Autodesk Fusion 360 part; units mm, degrees
(part 3 of 4)
sketch "Sketch6" plane through (0, 0, 4.8) normal (0, 0, 1) x (-1, 0, 0)
  circle A0 centre (64.2941, -62.4) radius 1.5
  circle A1 centre (64.2941, 62.4) radius 1.5
  circle A2 centre (97.2941, -62.4) radius 1.5
  circle A3 centre (97.2941, 62.4) radius 1.5
  circle A4 centre (1.7941, -104.2) radius 6.1
  line L0 (15.4941, 111.4) -> (41.8941, 111.4)
  arc A5 (45.5941, 107.7) -> (41.8941, 111.4) centre (41.8941, 107.7) ccw
  line L1 (45.5941, 107.7) -> (45.5941, 100.7)
  arc A6 (41.8941, 97) -> (45.5941, 100.7) centre (41.8941, 100.7) ccw
  line L2 (41.8941, 97) -> (15.4941, 97)
  arc A7 (11.7941, 100.7) -> (15.4941, 97) centre (15.4941, 100.7) ccw
  line L3 (11.7941, 100.7) -> (11.7941, 107.7)
  arc A8 (15.4941, 111.4) -> (11.7941, 107.7) centre (15.4941, 107.7) ccw
  line L4 (15.4941, -97) -> (41.8941, -97)
  arc A9 (45.5941, -100.7) -> (41.8941, -97) centre (41.8941, -100.7) ccw
  line L5 (45.5941, -100.7) -> (45.5941, -107.7)
  arc A10 (41.8941, -111.4) -> (45.5941, -107.7) centre (41.8941, -107.7) ccw
  line L6 (41.8941, -111.4) -> (15.4941, -111.4)
  arc A11 (11.7941, -107.7) -> (15.4941, -111.4) centre (15.4941, -107.7) ccw
  line L7 (11.7941, -107.7) -> (11.7941, -100.7)
  arc A12 (15.4941, -97) -> (11.7941, -100.7) centre (15.4941, -100.7) ccw
  circle A13 centre (45.4941, 42.5) radius 1.5
  arc A14 (94.6728, -10) -> (96.7941, -7.8787) centre (95.7335, -8.9393) ccw
  line L8 (94.6728, -10) -> (94.1155, -10)
  arc A15 (91.9941, -7.8787) -> (94.1155, -10) centre (93.0548, -8.9393) ccw
  line L9 (91.9941, -7.8787) -> (91.9941, 7.8787)
  arc A16 (94.1155, 10) -> (91.9941, 7.8787) centre (93.0548, 8.9393) ccw
  line L10 (94.1155, 10) -> (94.6728, 10)
  arc A17 (96.7941, 7.8787) -> (94.6728, 10) centre (95.7335, 8.9393) ccw
  line L11 (96.7941, 7.8787) -> (96.7941, -7.8787)
  arc A18 (39.8728, -10) -> (41.9941, -7.8787) centre (40.9335, -8.9393) ccw
  line L12 (39.8728, -10) -> (39.3155, -10)
  arc A19 (37.1941, -7.8787) -> (39.3155, -10) centre (38.2548, -8.9393) ccw
  line L13 (37.1941, -7.8787) -> (37.1941, 7.8787)
  arc A20 (39.3155, 10) -> (37.1941, 7.8787) centre (38.2548, 8.9393) ccw
  line L14 (39.3155, 10) -> (39.8728, 10)
  arc A21 (41.9941, 7.8787) -> (39.8728, 10) centre (40.9335, 8.9393) ccw
  line L15 (41.9941, 7.8787) -> (41.9941, -7.8787)
  circle A22 centre (-123.5112, 37.2289) radius 1.5
  circle A23 centre (64.5, 111.7173) radius 1.5
  arc A24 (-55.2202, 79.8868) -> (-55.9967, 76.9891) centre (-55.6084, 78.438) ccw
  line L16 (-55.2202, 79.8868) -> (-41.5739, 87.7655)
  arc A25 (-38.6762, 86.9891) -> (-41.5739, 87.7655) centre (-40.125, 87.3773) ccw
  line L17 (-38.6762, 86.9891) -> (-38.3975, 86.5064)
  arc A26 (-39.1739, 83.6086) -> (-38.3975, 86.5064) centre (-38.7857, 85.0575) ccw
  line L18 (-39.1739, 83.6086) -> (-52.8202, 75.7299)
  arc A27 (-55.718, 76.5064) -> (-52.8202, 75.7299) centre (-54.2691, 76.1181) ccw
  line L19 (-55.718, 76.5064) -> (-55.9967, 76.9891)
  circle A28 centre (-123.5112, -37.2289) radius 1.5
  circle A29 centre (64.5, -111.7173) radius 1.5
  arc A30 (-11.2762, 39.5309) -> (-14.1739, 40.3073) centre (-12.725, 39.9191) ccw
  line L20 (-11.2762, 39.5309) -> (-10.9975, 39.0482)
  arc A31 (-11.7739, 36.1504) -> (-10.9975, 39.0482) centre (-11.3857, 37.5993) ccw
  line L21 (-11.7739, 36.1504) -> (-25.4202, 28.2717)
  arc A32 (-28.318, 29.0482) -> (-25.4202, 28.2717) centre (-26.8691, 28.66) ccw
  line L22 (-28.318, 29.0482) -> (-28.5967, 29.5309)
  arc A33 (-27.8202, 32.4286) -> (-28.5967, 29.5309) centre (-28.2084, 30.9798) ccw
  line L23 (-27.8202, 32.4286) -> (-14.1739, 40.3073)
  arc A34 (-10.9975, -39.0482) -> (-11.7739, -36.1504) centre (-11.3857, -37.5993) ccw
  line L24 (-10.9975, -39.0482) -> (-11.2762, -39.5309)
  arc A35 (-14.1739, -40.3073) -> (-11.2762, -39.5309) centre (-12.725, -39.9191) ccw
  line L25 (-14.1739, -40.3073) -> (-27.8202, -32.4286)
  arc A36 (-28.5967, -29.5309) -> (-27.8202, -32.4286) centre (-28.2084, -30.9798) ccw
  line L26 (-28.5967, -29.5309) -> (-28.318, -29.0482)
  arc A37 (-25.4202, -28.2717) -> (-28.318, -29.0482) centre (-26.8691, -28.66) ccw
  line L27 (-25.4202, -28.2717) -> (-11.7739, -36.1504)
  arc A38 (-52.8202, -75.7299) -> (-55.718, -76.5064) centre (-54.2691, -76.1181) ccw
  line L28 (-52.8202, -75.7299) -> (-39.1739, -83.6086)
  arc A39 (-38.3975, -86.5064) -> (-39.1739, -83.6086) centre (-38.7857, -85.0575) ccw
  line L29 (-38.3975, -86.5064) -> (-38.6762, -86.9891)
  arc A40 (-41.5739, -87.7655) -> (-38.6762, -86.9891) centre (-40.125, -87.3773) ccw
  line L30 (-41.5739, -87.7655) -> (-55.2202, -79.8868)
  arc A41 (-55.9967, -76.9891) -> (-55.2202, -79.8868) centre (-55.6084, -78.438) ccw
  line L31 (-55.9967, -76.9891) -> (-55.718, -76.5064)
  circle A42 centre (45.4941, -42.5) radius 1.5
  line L32 (-42.1213, -25.5) -> (-109.5263, -25.5)
  arc A43 (-109.5263, -25.5) -> (-110.7763, -25.8349) centre (-109.5263, -28) ccw
  line L33 (-110.7763, -25.8349) -> (-125.9451, -34.5927)
  arc A44 (-125.9451, -34.5927) -> (-127.0931, -37.4646) centre (-124.6951, -36.7577) ccw
  arc A45 (-127.0931, -37.4646) -> (-89.0244, -98.1371) centre (0, 0) ccw
  arc A46 (-89.0244, -98.1371) -> (-85.1797, -97.5355) centre (-87.3447, -96.2855) ccw
  line L34 (-85.1797, -97.5355) -> (-74.6084, -79.2255)
  arc A47 (-71.7106, -78.449) -> (-74.6084, -79.2255) centre (-73.1595, -78.8372) ccw
  line L35 (-71.7106, -78.449) -> (-32.0836, -101.3277)
  arc A48 (-31.3071, -104.2255) -> (-32.0836, -101.3277) centre (-31.6953, -102.7766) ccw
  line L36 (-31.3071, -104.2255) -> (-41.8784, -122.5355)
  arc A49 (-41.8784, -122.5355) -> (-40.477, -126.166) centre (-39.7133, -123.7855) ccw
  arc A50 (-40.477, -126.166) -> (129.5015, -28.0288) centre (0, 0) ccw
  arc A51 (129.5015, -28.0288) -> (127.0581, -25) centre (127.0581, -27.5) ccw
  line L37 (127.0581, -25) -> (105.9155, -25)
  arc A52 (103.7941, -22.8787) -> (105.9155, -25) centre (104.8548, -23.9393) ccw
  line L38 (103.7941, -22.8787) -> (103.7941, 22.8787)
  arc A53 (105.9155, 25) -> (103.7941, 22.8787) centre (104.8548, 23.9393) ccw
  line L39 (105.9155, 25) -> (127.0581, 25)
  arc A54 (127.0581, 25) -> (129.5015, 28.0288) centre (127.0581, 27.5) ccw
  arc A55 (129.5015, 28.0288) -> (-40.477, 126.166) centre (0, 0) ccw
  arc A56 (-40.477, 126.166) -> (-41.8784, 122.5355) centre (-39.7133, 123.7855) ccw
  line L40 (-41.8784, 122.5355) -> (-31.3071, 104.2255)
  arc A57 (-32.0836, 101.3277) -> (-31.3071, 104.2255) centre (-31.6953, 102.7766) ccw
  line L41 (-32.0836, 101.3277) -> (-71.7106, 78.449)
  arc A58 (-74.6084, 79.2255) -> (-71.7106, 78.449) centre (-73.1595, 78.8372) ccw
  line L42 (-74.6084, 79.2255) -> (-85.1797, 97.5355)
  arc A59 (-85.1797, 97.5355) -> (-89.0244, 98.1371) centre (-87.3447, 96.2855) ccw
  arc A60 (-89.0244, 98.1371) -> (-127.0931, 37.4646) centre (0, 0) ccw
  arc A61 (-127.0931, 37.4646) -> (-125.9451, 34.5927) centre (-124.6951, 36.7577) ccw
  line L43 (-125.9451, 34.5927) -> (-110.7763, 25.8349)
  arc A62 (-110.7763, 25.8349) -> (-109.5263, 25.5) centre (-109.5263, 28) ccw
  line L44 (-109.5263, 25.5) -> (-42.1213, 25.5)
  arc A63 (-40, 23.3787) -> (-42.1213, 25.5) centre (-41.0607, 24.4393) ccw
  line L45 (-40, 23.3787) -> (-40, 20.8)
  arc A64 (-40, 20.8) -> (-37.5, 18.3) centre (-37.5, 20.8) ccw
  line L46 (-37.5, 18.3) -> (-34.1213, 18.3)
  arc A65 (-32, 16.1787) -> (-34.1213, 18.3) centre (-33.0607, 17.2393) ccw
  line L47 (-32, 16.1787) -> (-32, -16.1787)
  arc A66 (-34.1213, -18.3) -> (-32, -16.1787) centre (-33.0607, -17.2393) ccw
  line L48 (-34.1213, -18.3) -> (-37.5, -18.3)
  arc A67 (-37.5, -18.3) -> (-40, -20.8) centre (-37.5, -20.8) ccw
  line L49 (-40, -20.8) -> (-40, -23.3787)
  arc A68 (-42.1213, -25.5) -> (-40, -23.3787) centre (-41.0607, -24.4393) ccw
  arc A69 (-40.477, -126.166) -> (129.5015, -28.0288) centre (0, 0) ccw
  line L50 (57.7941, -64.8) -> (103.7941, -64.8)
  line L51 (57.7941, -58.1213) -> (57.7941, -83.8787)
  arc A70 (129.5015, 28.0288) -> (-40.477, 126.166) centre (0, 0) ccw
  line L52 (57.7941, 64.8) -> (103.7941, 64.8)
  line L53 (57.7941, 58.1213) -> (57.7941, 83.8787)
  line L54 (95.1844, -72.8) -> (67.2941, -72.8)
  line L55 (65.7941, -74.3) -> (65.7941, -100.26)
  arc A71 (68.1301, -101.5054) -> (96.3668, -75.223) centre (0, 0) ccw
  arc A72 (67.2941, -72.8) -> (65.7941, -74.3) centre (67.2941, -74.3) ccw
  arc A73 (65.7941, -100.26) -> (68.1301, -101.5054) centre (67.2941, -100.26) ccw
  arc A74 (96.3668, -75.223) -> (95.1844, -72.8) centre (95.1844, -74.3) ccw
  line L56 (95.1844, 72.8) -> (67.2941, 72.8)
  line L57 (65.7941, 74.3) -> (65.7941, 100.26)
  arc A75 (96.3668, 75.223) -> (68.1301, 101.5054) centre (0, 0) ccw
  arc A76 (65.7941, 74.3) -> (67.2941, 72.8) centre (67.2941, 74.3) ccw
  arc A77 (95.1844, 72.8) -> (96.3668, 75.223) centre (95.1844, 74.3) ccw
  arc A78 (68.1301, 101.5054) -> (65.7941, 100.26) centre (67.2941, 100.26) ccw
  circle A79 centre (-94.9024, 87.3758) radius 1.5
  circle A80 centre (123.1209, -38.5) radius 1.5
  circle A81 centre (123.1209, 38.5) radius 1.5
  circle A82 centre (-28.2185, 125.8758) radius 1.5
  circle A83 centre (-94.9024, -87.3758) radius 1.5
  circle A84 centre (-28.2185, -125.8758) radius 1.5
  dimension "d304" = 8
  dimension "d305" = 8
  dimension "d306" = 122.25
  dimension "d307" = 1.5
  dimension "d308" = 1.5
  dimension "d309" = 1.5
  dimension "d310" = 8
  dimension "d311" = 8
  dimension "d312" = 122.25
  dimension "d313" = 1.5
  dimension "d314" = 1.5
  dimension "d315" = 1.5
  constraint perpendicular L51 L54
  constraint perpendicular L54 L55
  constraint coincident A45.centre A50.centre
  constraint tangent L54 A72
  constraint tangent L55 A72
  constraint tangent A71 A73
  constraint tangent L55 A73
  constraint tangent A71 A74
  constraint tangent L54 A74
  constraint perpendicular L53 L56
  constraint perpendicular L56 L57
  constraint tangent L56 A76
  constraint tangent L57 A76
  constraint tangent A75 A77
  constraint tangent L56 A77
  constraint tangent A75 A78
  constraint tangent L57 A78
  measures "d304" distance of L50 L54
  measures "d305" distance of L51 L55
  measures "d306" radius of A71
  measures "d307" radius of A72
  measures "d308" radius of A73
  measures "d309" radius of A74
  measures "d310" distance of L52 L56
  measures "d311" distance of L53 L57
  measures "d312" radius of A75
  measures "d313" radius of A76
  measures "d314" radius of A77
  measures "d315" radius of A78
extrude "Extrude9" cut sketch "Sketch6" against normal through all contours L54 L55 A71 A72 A73 A74 | L56 L57 A75 A76 A77 A78
sketch "Sketch7" plane through (0, 0, 4.8) normal (0, 0, 1) x (-1, 0, 0)
  line L0 (11.7941, 92) -> (48.7941, 92)
  line L1 (11.7941, 89.8787) -> (11.7941, 58.1213)
  line L2 (57.7941, 58.1213) -> (57.7941, 83.8787)
  line L3 (48.7941, 56) -> (11.7941, 56)
  line L4 (11.7941, -56) -> (48.7941, -56)
  line L5 (11.7941, -92) -> (11.7941, -56)
  line L6 (13.9155, -92) -> (46.6728, -92)
  line L7 (57.7941, -86) -> (57.7941, -56)
  line L8 (16.2941, 92) -> (53.2941, 92) construction
  line L9 (53.2941, 92) -> (53.2941, 56) construction
  line L10 (53.2941, 56) -> (16.2941, 56) construction
  line L11 (16.2941, 56) -> (16.2941, 92) construction
  line L12 (48.7941, 92) -> (48.7941, 56) construction
  line L13 (57.7941, 86) -> (48.7941, 86) construction
  line L14 (11.7941, 89) -> (57.7941, 89) construction
  line L15 (57.7941, 89) -> (57.7941, 59) construction
  line L16 (57.7941, 59) -> (11.7941, 59) construction
  line L17 (11.7941, 59) -> (11.7941, 89) construction
  line L18 (16.2941, 92) -> (17.3548, 90.9393) construction
  line L19 (11.7941, 89) -> (12.8548, 87.9393) construction
  line L20 (53.2941, 92) -> (52.2335, 90.9393) construction
  line L21 (57.7941, 89) -> (56.7335, 87.9393) construction
  line L22 (57.7941, 59) -> (56.7335, 60.0607) construction
  line L23 (53.2941, 56) -> (52.2335, 57.0607) construction
  line L24 (16.2941, 56) -> (17.3548, 57.0607) construction
  line L25 (11.7941, 59) -> (12.8548, 60.0607) construction
  arc A0 (18.4155, 92) -> (16.2941, 89.8787) centre (17.3548, 90.9393) ccw
  arc A1 (16.2941, 89.8787) -> (18.4155, 92) centre (17.3548, 90.9393) ccw construction
  arc A2 (13.9155, 89) -> (11.7941, 86.8787) centre (12.8548, 87.9393) ccw
  arc A3 (11.7941, 86.8787) -> (13.9155, 89) centre (12.8548, 87.9393) ccw construction
  arc A4 (53.2941, 89.8787) -> (51.1728, 92) centre (52.2335, 90.9393) ccw
  arc A5 (51.1728, 92) -> (53.2941, 89.8787) centre (52.2335, 90.9393) ccw construction
  arc A6 (57.7941, 86.8787) -> (55.6728, 89) centre (56.7335, 87.9393) ccw
  arc A7 (55.6728, 89) -> (57.7941, 86.8787) centre (56.7335, 87.9393) ccw construction
  arc A8 (55.6728, 59) -> (57.7941, 61.1213) centre (56.7335, 60.0607) ccw
  arc A9 (57.7941, 61.1213) -> (55.6728, 59) centre (56.7335, 60.0607) ccw construction
  arc A10 (51.1728, 56) -> (53.2941, 58.1213) centre (52.2335, 57.0607) ccw
  arc A11 (53.2941, 58.1213) -> (51.1728, 56) centre (52.2335, 57.0607) ccw construction
  arc A12 (16.2941, 58.1213) -> (18.4155, 56) centre (17.3548, 57.0607) ccw
  arc A13 (18.4155, 56) -> (16.2941, 58.1213) centre (17.3548, 57.0607) ccw construction
  arc A14 (11.7941, 61.1213) -> (13.9155, 59) centre (12.8548, 60.0607) ccw
  arc A15 (13.9155, 59) -> (11.7941, 61.1213) centre (12.8548, 60.0607) ccw construction
  line L26 (53.2941, 58.1213) -> (53.2941, 59)
  line L27 (53.2941, 59) -> (55.6728, 59)
  line L28 (51.1728, 56) -> (18.4155, 56)
  line L29 (16.2941, 58.1213) -> (16.2941, 59)
  line L30 (16.2941, 59) -> (13.9155, 59)
  line L31 (11.7941, 61.1213) -> (11.7941, 86.8787)
  line L32 (13.9155, 89) -> (16.2941, 89)
  line L33 (16.2941, 89) -> (16.2941, 89.8787)
  line L34 (18.4155, 92) -> (51.1728, 92)
  line L35 (53.2941, 89.8787) -> (53.2941, 89)
  line L36 (53.2941, 89) -> (55.6728, 89)
  line L37 (57.7941, 86.8787) -> (57.7941, 61.1213)
  line L38 (11.7941, -59) -> (57.7941, -59) construction
  line L39 (57.7941, -59) -> (57.7941, -89) construction
  line L40 (57.7941, -89) -> (11.7941, -89) construction
  line L41 (11.7941, -89) -> (11.7941, -59) construction
  line L42 (16.2941, -56) -> (53.2941, -56) construction
  line L43 (53.2941, -56) -> (53.2941, -92) construction
  line L44 (53.2941, -92) -> (16.2941, -92) construction
  line L45 (16.2941, -92) -> (16.2941, -56) construction
  line L46 (11.7941, -89) -> (12.8548, -87.9393) construction
  line L47 (16.2941, -92) -> (17.3548, -90.9393) construction
  line L48 (53.2941, -92) -> (52.2335, -90.9393) construction
  line L49 (57.7941, -89) -> (56.7335, -87.9393) construction
  line L50 (57.7941, -59) -> (56.7335, -60.0607) construction
  line L51 (53.2941, -56) -> (52.2335, -57.0607) construction
  line L52 (16.2941, -56) -> (17.3548, -57.0607) construction
  line L53 (11.7941, -59) -> (12.8548, -60.0607) construction
  arc A16 (18.4155, -56) -> (16.2941, -58.1213) centre (17.3548, -57.0607) ccw
  arc A17 (16.2941, -58.1213) -> (18.4155, -56) centre (17.3548, -57.0607) ccw construction
  arc A18 (13.9155, -59) -> (11.7941, -61.1213) centre (12.8548, -60.0607) ccw
  arc A19 (11.7941, -61.1213) -> (13.9155, -59) centre (12.8548, -60.0607) ccw construction
  arc A20 (53.2941, -58.1213) -> (51.1728, -56) centre (52.2335, -57.0607) ccw
  arc A21 (51.1728, -56) -> (53.2941, -58.1213) centre (52.2335, -57.0607) ccw construction
  arc A22 (57.7941, -61.1213) -> (55.6728, -59) centre (56.7335, -60.0607) ccw
  arc A23 (55.6728, -59) -> (57.7941, -61.1213) centre (56.7335, -60.0607) ccw construction
  arc A24 (55.6728, -89) -> (57.7941, -86.8787) centre (56.7335, -87.9393) ccw
  arc A25 (57.7941, -86.8787) -> (55.6728, -89) centre (56.7335, -87.9393) ccw construction
  arc A26 (51.1728, -92) -> (53.2941, -89.8787) centre (52.2335, -90.9393) ccw
  arc A27 (53.2941, -89.8787) -> (51.1728, -92) centre (52.2335, -90.9393) ccw construction
  arc A28 (16.2941, -89.8787) -> (18.4155, -92) centre (17.3548, -90.9393) ccw
  arc A29 (18.4155, -92) -> (16.2941, -89.8787) centre (17.3548, -90.9393) ccw construction
  arc A30 (11.7941, -86.8787) -> (13.9155, -89) centre (12.8548, -87.9393) ccw
  arc A31 (13.9155, -89) -> (11.7941, -86.8787) centre (12.8548, -87.9393) ccw construction
  line L54 (18.4155, -56) -> (51.1728, -56)
  line L55 (11.7941, -61.1213) -> (11.7941, -86.8787)
  line L56 (57.7941, -61.1213) -> (57.7941, -86.8787)
  line L57 (51.1728, -92) -> (18.4155, -92)
  line L58 (13.9155, -89) -> (16.2941, -89)
  line L59 (16.2941, -89) -> (16.2941, -89.8787)
  line L60 (53.2941, -89.8787) -> (53.2941, -89)
  line L61 (53.2941, -89) -> (55.6728, -89)
  line L62 (55.6728, -59) -> (53.2941, -59)
  line L63 (53.2941, -58.1213) -> (53.2941, -59)
  line L64 (13.9155, -59) -> (16.2941, -59)
  line L65 (16.2941, -59) -> (16.2941, -58.1213)
  dimension "d319" = 37
  dimension "d322" = 4.5
  dimension "d323" = 30
  dimension "d324" = 3
  dimension "d325" = 36
  dimension "d326" = 46
  dimension "d327" = 1.5
  dimension "d328" = 1.5
  dimension "d329" = 1.5
  dimension "d330" = 1.5
  dimension "d331" = 1.5
  dimension "d332" = 1.5
  dimension "d333" = 1.5
  dimension "d334" = 1.5
  dimension "d335" = 45
  dimension "d336" = 45
  dimension "d337" = 45
  dimension "d338" = 45
  dimension "d339" = 45
  dimension "d340" = 45
  dimension "d341" = 45
  dimension "d342" = 45
  dimension "d343" = 36
  dimension "d344" = 30
  dimension "d345" = 3
  dimension "d346" = 37
  dimension "d347" = 4.5
  dimension "d349" = 1.5
  dimension "d350" = 1.5
  dimension "d351" = 1.5
  dimension "d352" = 1.5
  dimension "d353" = 1.5
  dimension "d354" = 1.5
  dimension "d355" = 1.5
  dimension "d356" = 1.5
  dimension "d357" = 45
  dimension "d358" = 45
  dimension "d359" = 45
  dimension "d360" = 45
  dimension "d361" = 45
  dimension "d362" = 45
  dimension "d363" = 45
  dimension "d364" = 45
  constraint horizontal L8
  constraint vertical L9
  constraint horizontal L10
  constraint vertical L11
  constraint coincident L0 L8.start
  constraint horizontal L14
  constraint vertical L15
  constraint horizontal L16
  constraint vertical L17
  constraint coincident L1 L14.start
  constraint coincident L22.end A8.centre
  constraint coincident L15.end A8
  constraint coincident L23.end A10.centre
  constraint coincident L9.end A10
  constraint coincident L24.end A12.centre
  constraint coincident L10.end A12
  constraint coincident L25.end A14.centre
  constraint coincident L16.end A14
  constraint coincident L20.end A4.centre
  constraint coincident L8.end A4
  constraint coincident L21.end A6.centre
  constraint coincident L14.end A6
  constraint coincident L19.end A2.centre
  constraint coincident L14.start A2
  constraint coincident L18.end A0.centre
  constraint coincident L8.start A0
  constraint coincident L11 A0.end
  constraint coincident L0 A0.start
  constraint concentric A0 A1
  constraint coincident L1 A2.end
  constraint coincident L14 A2.start
  constraint concentric A2 A3
  constraint coincident L8 A4.end
  constraint coincident L9 A4.start
  constraint concentric A4 A5
  constraint coincident L14 A6.end
  constraint coincident L15 A6.start
  constraint concentric A6 A7
  constraint coincident L2 A8.end
  constraint coincident L16 A8.start
  constraint concentric A8 A9
  constraint coincident L9 A10.end
  constraint coincident L10 A10.start
  constraint concentric A10 A11
  constraint coincident L3 A12.end
  constraint coincident L11 A12.start
  constraint concentric A12 A13
  constraint coincident L16 A14.end
  constraint coincident L1 A14.start
  constraint concentric A14 A15
  constraint coincident L9 L26.end
  constraint coincident L16 L26.end
  constraint coincident L16 L29.end
  constraint coincident L11 L29.end
  constraint coincident L14 L32.end
  constraint coincident L11 L32.end
  constraint coincident L14 L35.end
  constraint coincident L9 L35.end
  constraint horizontal L38
  constraint vertical L39
  constraint horizontal L40
  constraint vertical L41
  constraint coincident L7 L39.end
  constraint coincident L5 L38.start
  constraint horizontal L42
  constraint vertical L43
  constraint horizontal L44
  constraint vertical L45
  constraint coincident L6 L43.end
  constraint coincident L4 L42.start
  constraint coincident L46.end A30.centre
  constraint coincident L40.end A30
  constraint coincident L47.end A28.centre
  constraint coincident L44.end A28
  constraint coincident L48.end A26.centre
  constraint coincident L43.end A26
  constraint coincident L49.end A24.centre
  constraint coincident L39.end A24
  constraint coincident L50.end A22.centre
  constraint coincident L38.end A22
  constraint coincident L51.end A20.centre
  constraint coincident L42.end A20
  constraint coincident L52.end A16.centre
  constraint coincident L42.start A16
  constraint coincident L53.end A18.centre
  constraint coincident L38.start A18
  constraint coincident L45 A16.end
  constraint coincident L4 A16.start
  constraint concentric A16 A17
  constraint coincident L5 A18.end
  constraint coincident L38 A18.start
  constraint concentric A18 A19
  constraint coincident L42 A20.end
  constraint coincident L43 A20.start
  constraint concentric A20 A21
  constraint coincident L38 A22.end
  constraint coincident L7 A22.start
  constraint concentric A22 A23
  constraint coincident L39 A24.end
  constraint coincident L40 A24.start
  constraint concentric A24 A25
  constraint coincident L43 A26.end
  constraint coincident L44 A26.start
  constraint concentric A26 A27
  constraint coincident L6 A28.end
  constraint coincident L45 A28.start
  constraint concentric A28 A29
  constraint coincident L40 A30.end
  constraint coincident L5 A30.start
  constraint concentric A30 A31
  constraint coincident L40 L58.end
  constraint coincident L45 L58.end
  constraint coincident L40 L60.end
  constraint coincident L43 L60.end
  constraint coincident L38 L62.end
  constraint coincident L43 L62.end
  constraint coincident L38 L64.end
  constraint coincident L45 L64.end
  measures "d319" distance of L8.start L8.end
  measures "d322" distance of L1 L11
  measures "d323" distance of L14.start L16.end
  measures "d324" distance of L8 L14
  measures "d325" distance of L8 L10
  measures "d326" distance of L15 L17
  measures "d327" distance of L8.start L18.end
  measures "d328" distance of L14.start L19.end
  measures "d329" distance of L8.end L20.end
  measures "d330" distance of L14.end L21.end
  measures "d331" distance of L15.end L22.end
  measures "d332" distance of L9.end L23.end
  measures "d333" distance of L10.end L24.end
  measures "d334" distance of L16.end L25.end
  measures "d335" angle of L10 L24
  measures "d336" angle of L16 L25
  measures "d337" angle of L14 L19
  measures "d338" angle of L8 L18
  measures "d339" angle of L8 L20
  measures "d340" angle of L14 L21
  measures "d341" angle of L10 L23
  measures "d342" angle of L16 L22
  measures "d343" distance of L42 L44
  measures "d344" distance of L38 L40
  measures "d345" distance of L38 L42
  measures "d346" distance of L43 L45
  measures "d347" distance of L39 L43
  measures "d349" distance of L40.end L46.end
  measures "d350" distance of L44.end L47.end
  measures "d351" distance of L43.end L48.end
  measures "d352" distance of L39.end L49.end
  measures "d353" distance of L38.end L50.end
  measures "d354" distance of L42.end L51.end
  measures "d355" distance of L42.start L52.end
  measures "d356" distance of L38.start L53.end
  measures "d357" angle of L38 L53
  measures "d358" angle of L42 L52
  measures "d359" angle of L42 L51
  measures "d360" angle of L38 L50
  measures "d361" angle of L40 L49
  measures "d362" angle of L44 L48
  measures "d363" angle of L44 L47
  measures "d364" angle of L40 L46
extrude "Extrude10" cut sketch "Sketch7" against normal through all contours L0 L1 L2 L3 A0 A2 A4 A6 A8 A10 A12 A14 L26 L27 L28 L29 L30 L31 L32 L33 L34 L35 L36 L37 | L0 A0 | L1 A2 | L1 A14 | L2 A8 | L3 A12 | L4 L5 L6 L7 A16 A18 A20 A22 A24 A26 A28 A30 L54 L55 L56 L57 L58 L59 L60 L61 L62 L63 L64 L65 | L4 A16 | L5 A18 | L5 A30 | L7 A22 | L6 A28
sketch "Sketch8" plane through (0, 0, 4.8) normal (0, 0, 1) x (-1, 0, 0)
  line L0 (57.7941, -61.1213) -> (57.7941, -86.8787)
  arc A0 (55.6728, -89) -> (57.7941, -86.8787) centre (56.7335, -87.9393) ccw
  line L1 (55.6728, -89) -> (53.2941, -89)
  line L2 (53.2941, -89) -> (53.2941, -89.8787)
  arc A1 (51.1728, -92) -> (53.2941, -89.8787) centre (52.2335, -90.9393) ccw
  line L3 (51.1728, -92) -> (18.4155, -92)
  arc A2 (16.2941, -89.8787) -> (18.4155, -92) centre (17.3548, -90.9393) ccw
  line L4 (16.2941, -89.8787) -> (16.2941, -89)
  line L5 (16.2941, -89) -> (13.9155, -89)
  arc A3 (11.7941, -86.8787) -> (13.9155, -89) centre (12.8548, -87.9393) ccw
  line L6 (11.7941, -86.8787) -> (11.7941, -61.1213)
  arc A4 (13.9155, -59) -> (11.7941, -61.1213) centre (12.8548, -60.0607) ccw
  line L7 (13.9155, -59) -> (16.2941, -59)
  line L8 (16.2941, -59) -> (16.2941, -58.1213)
  arc A5 (18.4155, -56) -> (16.2941, -58.1213) centre (17.3548, -57.0607) ccw
  line L9 (18.4155, -56) -> (51.1728, -56)
  arc A6 (53.2941, -58.1213) -> (51.1728, -56) centre (52.2335, -57.0607) ccw
  line L10 (53.2941, -58.1213) -> (53.2941, -59)
  line L11 (53.2941, -59) -> (55.6728, -59)
  arc A7 (57.7941, -61.1213) -> (55.6728, -59) centre (56.7335, -60.0607) ccw
  line L12 (51.1728, 56) -> (18.4155, 56)
  arc A8 (16.2941, 58.1213) -> (18.4155, 56) centre (17.3548, 57.0607) ccw
  line L13 (16.2941, 58.1213) -> (16.2941, 59)
  line L14 (16.2941, 59) -> (13.9155, 59)
  arc A9 (11.7941, 61.1213) -> (13.9155, 59) centre (12.8548, 60.0607) ccw
  line L15 (11.7941, 61.1213) -> (11.7941, 86.8787)
  arc A10 (13.9155, 89) -> (11.7941, 86.8787) centre (12.8548, 87.9393) ccw
  line L16 (13.9155, 89) -> (16.2941, 89)
  line L17 (16.2941, 89) -> (16.2941, 89.8787)
  arc A11 (18.4155, 92) -> (16.2941, 89.8787) centre (17.3548, 90.9393) ccw
  line L18 (18.4155, 92) -> (51.1728, 92)
  arc A12 (53.2941, 89.8787) -> (51.1728, 92) centre (52.2335, 90.9393) ccw
  line L19 (53.2941, 89.8787) -> (53.2941, 89)
  line L20 (53.2941, 89) -> (55.6728, 89)
  arc A13 (57.7941, 86.8787) -> (55.6728, 89) centre (56.7335, 87.9393) ccw
  line L21 (57.7941, 86.8787) -> (57.7941, 61.1213)
  arc A14 (55.6728, 59) -> (57.7941, 61.1213) centre (56.7335, 60.0607) ccw
  line L22 (55.6728, 59) -> (53.2941, 59)
  line L23 (53.2941, 59) -> (53.2941, 58.1213)
  arc A15 (51.1728, 56) -> (53.2941, 58.1213) centre (52.2335, 57.0607) ccw
  arc A16 (65.7941, 74.3) -> (67.2941, 72.8) centre (67.2941, 74.3) ccw
  line L24 (65.7941, 74.3) -> (65.7941, 100.26)
  arc A17 (68.1301, 101.5054) -> (65.7941, 100.26) centre (67.2941, 100.26) ccw
  arc A18 (96.3668, 75.223) -> (68.1301, 101.5054) centre (0, 0) ccw
  arc A19 (95.1844, 72.8) -> (96.3668, 75.223) centre (95.1844, 74.3) ccw
  line L25 (95.1844, 72.8) -> (67.2941, 72.8)
  arc A20 (65.7941, -100.26) -> (68.1301, -101.5054) centre (67.2941, -100.26) ccw
  line L26 (65.7941, -100.26) -> (65.7941, -74.3)
  arc A21 (67.2941, -72.8) -> (65.7941, -74.3) centre (67.2941, -74.3) ccw
  line L27 (67.2941, -72.8) -> (95.1844, -72.8)
  arc A22 (96.3668, -75.223) -> (95.1844, -72.8) centre (95.1844, -74.3) ccw
  arc A23 (68.1301, -101.5054) -> (96.3668, -75.223) centre (0, 0) ccw
  circle A24 centre (64.2941, -62.4) radius 1.5
  circle A25 centre (64.2941, 62.4) radius 1.5
  circle A26 centre (97.2941, -62.4) radius 1.5
  circle A27 centre (97.2941, 62.4) radius 1.5
  circle A28 centre (1.7941, -104.2) radius 6.1
  line L28 (15.4941, 111.4) -> (41.8941, 111.4)
  arc A29 (45.5941, 107.7) -> (41.8941, 111.4) centre (41.8941, 107.7) ccw
  line L29 (45.5941, 107.7) -> (45.5941, 100.7)
  arc A30 (41.8941, 97) -> (45.5941, 100.7) centre (41.8941, 100.7) ccw
  line L30 (41.8941, 97) -> (15.4941, 97)
  arc A31 (11.7941, 100.7) -> (15.4941, 97) centre (15.4941, 100.7) ccw
  line L31 (11.7941, 100.7) -> (11.7941, 107.7)
  arc A32 (15.4941, 111.4) -> (11.7941, 107.7) centre (15.4941, 107.7) ccw
  line L32 (15.4941, -97) -> (41.8941, -97)
  arc A33 (45.5941, -100.7) -> (41.8941, -97) centre (41.8941, -100.7) ccw
  line L33 (45.5941, -100.7) -> (45.5941, -107.7)
  arc A34 (41.8941, -111.4) -> (45.5941, -107.7) centre (41.8941, -107.7) ccw
  line L34 (41.8941, -111.4) -> (15.4941, -111.4)
  arc A35 (11.7941, -107.7) -> (15.4941, -111.4) centre (15.4941, -107.7) ccw
  line L35 (11.7941, -107.7) -> (11.7941, -100.7)
  arc A36 (15.4941, -97) -> (11.7941, -100.7) centre (15.4941, -100.7) ccw
  circle A37 centre (64.5, 111.7173) radius 1.5
  arc A38 (-55.2202, 79.8868) -> (-55.9967, 76.9891) centre (-55.6084, 78.438) ccw
  line L36 (-55.2202, 79.8868) -> (-41.5739, 87.7655)
  arc A39 (-38.6762, 86.9891) -> (-41.5739, 87.7655) centre (-40.125, 87.3773) ccw
  line L37 (-38.6762, 86.9891) -> (-38.3975, 86.5064)
  arc A40 (-39.1739, 83.6086) -> (-38.3975, 86.5064) centre (-38.7857, 85.0575) ccw
  line L38 (-39.1739, 83.6086) -> (-52.8202, 75.7299)
  arc A41 (-55.718, 76.5064) -> (-52.8202, 75.7299) centre (-54.2691, 76.1181) ccw
  line L39 (-55.718, 76.5064) -> (-55.9967, 76.9891)
  circle A42 centre (-123.5112, -37.2289) radius 1.5
  circle A43 centre (-123.5112, 37.2289) radius 1.5
  circle A44 centre (64.5, -111.7173) radius 1.5
  arc A45 (-11.2762, 39.5309) -> (-14.1739, 40.3073) centre (-12.725, 39.9191) ccw
  line L40 (-11.2762, 39.5309) -> (-10.9975, 39.0482)
  arc A46 (-11.7739, 36.1504) -> (-10.9975, 39.0482) centre (-11.3857, 37.5993) ccw
  line L41 (-11.7739, 36.1504) -> (-25.4202, 28.2717)
  arc A47 (-28.318, 29.0482) -> (-25.4202, 28.2717) centre (-26.8691, 28.66) ccw
  line L42 (-28.318, 29.0482) -> (-28.5967, 29.5309)
  arc A48 (-27.8202, 32.4286) -> (-28.5967, 29.5309) centre (-28.2084, 30.9798) ccw
  line L43 (-27.8202, 32.4286) -> (-14.1739, 40.3073)
  arc A49 (-10.9975, -39.0482) -> (-11.7739, -36.1504) centre (-11.3857, -37.5993) ccw
  line L44 (-10.9975, -39.0482) -> (-11.2762, -39.5309)
  arc A50 (-14.1739, -40.3073) -> (-11.2762, -39.5309) centre (-12.725, -39.9191) ccw
  line L45 (-14.1739, -40.3073) -> (-27.8202, -32.4286)
  arc A51 (-28.5967, -29.5309) -> (-27.8202, -32.4286) centre (-28.2084, -30.9798) ccw
  line L46 (-28.5967, -29.5309) -> (-28.318, -29.0482)
  arc A52 (-25.4202, -28.2717) -> (-28.318, -29.0482) centre (-26.8691, -28.66) ccw
  line L47 (-25.4202, -28.2717) -> (-11.7739, -36.1504)
  circle A53 centre (45.4941, 42.5) radius 1.5
  arc A54 (-52.8202, -75.7299) -> (-55.718, -76.5064) centre (-54.2691, -76.1181) ccw
  line L48 (-52.8202, -75.7299) -> (-39.1739, -83.6086)
  arc A55 (-38.3975, -86.5064) -> (-39.1739, -83.6086) centre (-38.7857, -85.0575) ccw
  line L49 (-38.3975, -86.5064) -> (-38.6762, -86.9891)
  arc A56 (-41.5739, -87.7655) -> (-38.6762, -86.9891) centre (-40.125, -87.3773) ccw
  line L50 (-41.5739, -87.7655) -> (-55.2202, -79.8868)
  arc A57 (-55.9967, -76.9891) -> (-55.2202, -79.8868) centre (-55.6084, -78.438) ccw
  line L51 (-55.9967, -76.9891) -> (-55.718, -76.5064)
  arc A58 (39.8728, -10) -> (41.9941, -7.8787) centre (40.9335, -8.9393) ccw
  line L52 (39.8728, -10) -> (39.3155, -10)
  arc A59 (37.1941, -7.8787) -> (39.3155, -10) centre (38.2548, -8.9393) ccw
  line L53 (37.1941, -7.8787) -> (37.1941, 7.8787)
  arc A60 (39.3155, 10) -> (37.1941, 7.8787) centre (38.2548, 8.9393) ccw
  line L54 (39.3155, 10) -> (39.8728, 10)
  arc A61 (41.9941, 7.8787) -> (39.8728, 10) centre (40.9335, 8.9393) ccw
  line L55 (41.9941, 7.8787) -> (41.9941, -7.8787)
  arc A62 (94.6728, -10) -> (96.7941, -7.8787) centre (95.7335, -8.9393) ccw
  line L56 (94.6728, -10) -> (94.1155, -10)
  arc A63 (91.9941, -7.8787) -> (94.1155, -10) centre (93.0548, -8.9393) ccw
  line L57 (91.9941, -7.8787) -> (91.9941, 7.8787)
  arc A64 (94.1155, 10) -> (91.9941, 7.8787) centre (93.0548, 8.9393) ccw
  line L58 (94.1155, 10) -> (94.6728, 10)
  arc A65 (96.7941, 7.8787) -> (94.6728, 10) centre (95.7335, 8.9393) ccw
  line L59 (96.7941, 7.8787) -> (96.7941, -7.8787)
  circle A66 centre (45.4941, -42.5) radius 1.5
  line L60 (-42.1213, -25.5) -> (-109.5263, -25.5)
  arc A67 (-109.5263, -25.5) -> (-110.7763, -25.8349) centre (-109.5263, -28) ccw
  line L61 (-110.7763, -25.8349) -> (-125.9451, -34.5927)
  arc A68 (-125.9451, -34.5927) -> (-127.0931, -37.4646) centre (-124.6951, -36.7577) ccw
  arc A69 (-127.0931, -37.4646) -> (-89.0244, -98.1371) centre (0, 0) ccw
  arc A70 (-89.0244, -98.1371) -> (-85.1797, -97.5355) centre (-87.3447, -96.2855) ccw
  line L62 (-85.1797, -97.5355) -> (-74.6084, -79.2255)
  arc A71 (-71.7106, -78.449) -> (-74.6084, -79.2255) centre (-73.1595, -78.8372) ccw
  line L63 (-71.7106, -78.449) -> (-32.0836, -101.3277)
  arc A72 (-31.3071, -104.2255) -> (-32.0836, -101.3277) centre (-31.6953, -102.7766) ccw
  line L64 (-31.3071, -104.2255) -> (-41.8784, -122.5355)
  arc A73 (-41.8784, -122.5355) -> (-40.477, -126.166) centre (-39.7133, -123.7855) ccw
  arc A74 (-40.477, -126.166) -> (129.5015, -28.0288) centre (0, 0) ccw
  arc A75 (129.5015, -28.0288) -> (127.0581, -25) centre (127.0581, -27.5) ccw
  line L65 (127.0581, -25) -> (105.9155, -25)
  arc A76 (103.7941, -22.8787) -> (105.9155, -25) centre (104.8548, -23.9393) ccw
  line L66 (103.7941, -22.8787) -> (103.7941, 22.8787)
  arc A77 (105.9155, 25) -> (103.7941, 22.8787) centre (104.8548, 23.9393) ccw
  line L67 (105.9155, 25) -> (127.0581, 25)
  arc A78 (127.0581, 25) -> (129.5015, 28.0288) centre (127.0581, 27.5) ccw
  arc A79 (129.5015, 28.0288) -> (-40.477, 126.166) centre (0, 0) ccw
  arc A80 (-40.477, 126.166) -> (-41.8784, 122.5355) centre (-39.7133, 123.7855) ccw
  line L68 (-41.8784, 122.5355) -> (-31.3071, 104.2255)
  arc A81 (-32.0836, 101.3277) -> (-31.3071, 104.2255) centre (-31.6953, 102.7766) ccw
  line L69 (-32.0836, 101.3277) -> (-71.7106, 78.449)
  arc A82 (-74.6084, 79.2255) -> (-71.7106, 78.449) centre (-73.1595, 78.8372) ccw
  line L70 (-74.6084, 79.2255) -> (-85.1797, 97.5355)
  arc A83 (-85.1797, 97.5355) -> (-89.0244, 98.1371) centre (-87.3447, 96.2855) ccw
  arc A84 (-89.0244, 98.1371) -> (-127.0931, 37.4646) centre (0, 0) ccw
  arc A85 (-127.0931, 37.4646) -> (-125.9451, 34.5927) centre (-124.6951, 36.7577) ccw
  line L71 (-125.9451, 34.5927) -> (-110.7763, 25.8349)
  arc A86 (-110.7763, 25.8349) -> (-109.5263, 25.5) centre (-109.5263, 28) ccw
  line L72 (-109.5263, 25.5) -> (-42.1213, 25.5)
  arc A87 (-40, 23.3787) -> (-42.1213, 25.5) centre (-41.0607, 24.4393) ccw
  line L73 (-40, 23.3787) -> (-40, 20.8)
  arc A88 (-40, 20.8) -> (-37.5, 18.3) centre (-37.5, 20.8) ccw
  line L74 (-37.5, 18.3) -> (-34.1213, 18.3)
  arc A89 (-32, 16.1787) -> (-34.1213, 18.3) centre (-33.0607, 17.2393) ccw
  line L75 (-32, 16.1787) -> (-32, -16.1787)
  arc A90 (-34.1213, -18.3) -> (-32, -16.1787) centre (-33.0607, -17.2393) ccw
  line L76 (-34.1213, -18.3) -> (-37.5, -18.3)
  arc A91 (-37.5, -18.3) -> (-40, -20.8) centre (-37.5, -20.8) ccw
  line L77 (-40, -20.8) -> (-40, -23.3787)
  arc A92 (-42.1213, -25.5) -> (-40, -23.3787) centre (-41.0607, -24.4393) ccw
  circle A93 centre (0, 0) radius 1.5
  circle A94 centre (-94.9024, 87.3758) radius 1.5
  circle A95 centre (123.1209, -38.5) radius 1.5
  circle A96 centre (123.1209, 38.5) radius 1.5
  circle A97 centre (-28.2185, 125.8758) radius 1.5
  circle A98 centre (-94.9024, -87.3758) radius 1.5
  circle A99 centre (-28.2185, -125.8758) radius 1.5
  dimension "d366" = 3
  constraint concentric A18 A93
  measures "d366" diameter of A93
extrude "Extrude11" cut sketch "Sketch8" against normal through all contours A93
sketch "Sketch9" plane through (0, 0, 4.8) normal (0, 0, 1) x (-1, 0, 0)
  circle A0 centre (0, 0) radius 1.5
  line L0 (57.7941, -61.1213) -> (57.7941, -86.8787)
  arc A1 (55.6728, -89) -> (57.7941, -86.8787) centre (56.7335, -87.9393) ccw
  line L1 (55.6728, -89) -> (53.2941, -89)
  line L2 (53.2941, -89) -> (53.2941, -89.8787)
  arc A2 (51.1728, -92) -> (53.2941, -89.8787) centre (52.2335, -90.9393) ccw
  line L3 (51.1728, -92) -> (18.4155, -92)
  arc A3 (16.2941, -89.8787) -> (18.4155, -92) centre (17.3548, -90.9393) ccw
  line L4 (16.2941, -89.8787) -> (16.2941, -89)
  line L5 (16.2941, -89) -> (13.9155, -89)
  arc A4 (11.7941, -86.8787) -> (13.9155, -89) centre (12.8548, -87.9393) ccw
  line L6 (11.7941, -86.8787) -> (11.7941, -61.1213)
  arc A5 (13.9155, -59) -> (11.7941, -61.1213) centre (12.8548, -60.0607) ccw
  line L7 (13.9155, -59) -> (16.2941, -59)
  line L8 (16.2941, -59) -> (16.2941, -58.1213)
  arc A6 (18.4155, -56) -> (16.2941, -58.1213) centre (17.3548, -57.0607) ccw
  line L9 (18.4155, -56) -> (51.1728, -56)
  arc A7 (53.2941, -58.1213) -> (51.1728, -56) centre (52.2335, -57.0607) ccw
  line L10 (53.2941, -58.1213) -> (53.2941, -59)
  line L11 (53.2941, -59) -> (55.6728, -59)
  arc A8 (57.7941, -61.1213) -> (55.6728, -59) centre (56.7335, -60.0607) ccw
  line L12 (51.1728, 56) -> (18.4155, 56)
  arc A9 (16.2941, 58.1213) -> (18.4155, 56) centre (17.3548, 57.0607) ccw
  line L13 (16.2941, 58.1213) -> (16.2941, 59)
  line L14 (16.2941, 59) -> (13.9155, 59)
  arc A10 (11.7941, 61.1213) -> (13.9155, 59) centre (12.8548, 60.0607) ccw
  line L15 (11.7941, 61.1213) -> (11.7941, 86.8787)
  arc A11 (13.9155, 89) -> (11.7941, 86.8787) centre (12.8548, 87.9393) ccw
  line L16 (13.9155, 89) -> (16.2941, 89)
  line L17 (16.2941, 89) -> (16.2941, 89.8787)
  arc A12 (18.4155, 92) -> (16.2941, 89.8787) centre (17.3548, 90.9393) ccw
  line L18 (18.4155, 92) -> (51.1728, 92)
  arc A13 (53.2941, 89.8787) -> (51.1728, 92) centre (52.2335, 90.9393) ccw
  line L19 (53.2941, 89.8787) -> (53.2941, 89)
  line L20 (53.2941, 89) -> (55.6728, 89)
  arc A14 (57.7941, 86.8787) -> (55.6728, 89) centre (56.7335, 87.9393) ccw
  line L21 (57.7941, 86.8787) -> (57.7941, 61.1213)
  arc A15 (55.6728, 59) -> (57.7941, 61.1213) centre (56.7335, 60.0607) ccw
  line L22 (55.6728, 59) -> (53.2941, 59)
  line L23 (53.2941, 59) -> (53.2941, 58.1213)
  arc A16 (51.1728, 56) -> (53.2941, 58.1213) centre (52.2335, 57.0607) ccw
  arc A17 (65.7941, 74.3) -> (67.2941, 72.8) centre (67.2941, 74.3) ccw
  line L24 (65.7941, 74.3) -> (65.7941, 100.26)
  arc A18 (68.1301, 101.5054) -> (65.7941, 100.26) centre (67.2941, 100.26) ccw
  arc A19 (96.3668, 75.223) -> (68.1301, 101.5054) centre (0, 0) ccw
  arc A20 (95.1844, 72.8) -> (96.3668, 75.223) centre (95.1844, 74.3) ccw
  line L25 (95.1844, 72.8) -> (67.2941, 72.8)
  arc A21 (65.7941, -100.26) -> (68.1301, -101.5054) centre (67.2941, -100.26) ccw
  line L26 (65.7941, -100.26) -> (65.7941, -74.3)
  arc A22 (67.2941, -72.8) -> (65.7941, -74.3) centre (67.2941, -74.3) ccw
  line L27 (67.2941, -72.8) -> (95.1844, -72.8)
  arc A23 (96.3668, -75.223) -> (95.1844, -72.8) centre (95.1844, -74.3) ccw
  arc A24 (68.1301, -101.5054) -> (96.3668, -75.223) centre (0, 0) ccw
  circle A25 centre (64.2941, -62.4) radius 1.5
  circle A26 centre (64.2941, 62.4) radius 1.5
  circle A27 centre (97.2941, -62.4) radius 1.5
  circle A28 centre (97.2941, 62.4) radius 1.5
  circle A29 centre (1.7941, -104.2) radius 6.1
  line L28 (15.4941, 111.4) -> (41.8941, 111.4)
  arc A30 (45.5941, 107.7) -> (41.8941, 111.4) centre (41.8941, 107.7) ccw
  line L29 (45.5941, 107.7) -> (45.5941, 100.7)
  arc A31 (41.8941, 97) -> (45.5941, 100.7) centre (41.8941, 100.7) ccw
  line L30 (41.8941, 97) -> (15.4941, 97)
  arc A32 (11.7941, 100.7) -> (15.4941, 97) centre (15.4941, 100.7) ccw
  line L31 (11.7941, 100.7) -> (11.7941, 107.7)
  arc A33 (15.4941, 111.4) -> (11.7941, 107.7) centre (15.4941, 107.7) ccw
  line L32 (15.4941, -97) -> (41.8941, -97)
  arc A34 (45.5941, -100.7) -> (41.8941, -97) centre (41.8941, -100.7) ccw
  line L33 (45.5941, -100.7) -> (45.5941, -107.7)
  arc A35 (41.8941, -111.4) -> (45.5941, -107.7) centre (41.8941, -107.7) ccw
  line L34 (41.8941, -111.4) -> (15.4941, -111.4)
  arc A36 (11.7941, -107.7) -> (15.4941, -111.4) centre (15.4941, -107.7) ccw
  line L35 (11.7941, -107.7) -> (11.7941, -100.7)
  arc A37 (15.4941, -97) -> (11.7941, -100.7) centre (15.4941, -100.7) ccw
  circle A38 centre (64.5, 111.7173) radius 1.5
  arc A39 (-55.2202, 79.8868) -> (-55.9967, 76.9891) centre (-55.6084, 78.438) ccw
  line L36 (-55.2202, 79.8868) -> (-41.5739, 87.7655)
  arc A40 (-38.6762, 86.9891) -> (-41.5739, 87.7655) centre (-40.125, 87.3773) ccw
  line L37 (-38.6762, 86.9891) -> (-38.3975, 86.5064)
  arc A41 (-39.1739, 83.6086) -> (-38.3975, 86.5064) centre (-38.7857, 85.0575) ccw
  line L38 (-39.1739, 83.6086) -> (-52.8202, 75.7299)
  arc A42 (-55.718, 76.5064) -> (-52.8202, 75.7299) centre (-54.2691, 76.1181) ccw
  line L39 (-55.718, 76.5064) -> (-55.9967, 76.9891)
  circle A43 centre (-123.5112, -37.2289) radius 1.5
  circle A44 centre (-123.5112, 37.2289) radius 1.5
  circle A45 centre (64.5, -111.7173) radius 1.5
  arc A46 (-11.2762, 39.5309) -> (-14.1739, 40.3073) centre (-12.725, 39.9191) ccw
  line L40 (-11.2762, 39.5309) -> (-10.9975, 39.0482)
  arc A47 (-11.7739, 36.1504) -> (-10.9975, 39.0482) centre (-11.3857, 37.5993) ccw
  line L41 (-11.7739, 36.1504) -> (-25.4202, 28.2717)
  arc A48 (-28.318, 29.0482) -> (-25.4202, 28.2717) centre (-26.8691, 28.66) ccw
  line L42 (-28.318, 29.0482) -> (-28.5967, 29.5309)
  arc A49 (-27.8202, 32.4286) -> (-28.5967, 29.5309) centre (-28.2084, 30.9798) ccw
  line L43 (-27.8202, 32.4286) -> (-14.1739, 40.3073)
  arc A50 (-10.9975, -39.0482) -> (-11.7739, -36.1504) centre (-11.3857, -37.5993) ccw
  line L44 (-10.9975, -39.0482) -> (-11.2762, -39.5309)
  arc A51 (-14.1739, -40.3073) -> (-11.2762, -39.5309) centre (-12.725, -39.9191) ccw
  line L45 (-14.1739, -40.3073) -> (-27.8202, -32.4286)
  arc A52 (-28.5967, -29.5309) -> (-27.8202, -32.4286) centre (-28.2084, -30.9798) ccw
  line L46 (-28.5967, -29.5309) -> (-28.318, -29.0482)
  arc A53 (-25.4202, -28.2717) -> (-28.318, -29.0482) centre (-26.8691, -28.66) ccw
  line L47 (-25.4202, -28.2717) -> (-11.7739, -36.1504)
  circle A54 centre (45.4941, 42.5) radius 1.5
  arc A55 (-52.8202, -75.7299) -> (-55.718, -76.5064) centre (-54.2691, -76.1181) ccw
  line L48 (-52.8202, -75.7299) -> (-39.1739, -83.6086)
  arc A56 (-38.3975, -86.5064) -> (-39.1739, -83.6086) centre (-38.7857, -85.0575) ccw
  line L49 (-38.3975, -86.5064) -> (-38.6762, -86.9891)
  arc A57 (-41.5739, -87.7655) -> (-38.6762, -86.9891) centre (-40.125, -87.3773) ccw
  line L50 (-41.5739, -87.7655) -> (-55.2202, -79.8868)
  arc A58 (-55.9967, -76.9891) -> (-55.2202, -79.8868) centre (-55.6084, -78.438) ccw
  line L51 (-55.9967, -76.9891) -> (-55.718, -76.5064)
  arc A59 (39.8728, -10) -> (41.9941, -7.8787) centre (40.9335, -8.9393) ccw
  line L52 (39.8728, -10) -> (39.3155, -10)
  arc A60 (37.1941, -7.8787) -> (39.3155, -10) centre (38.2548, -8.9393) ccw
  line L53 (37.1941, -7.8787) -> (37.1941, 7.8787)
  arc A61 (39.3155, 10) -> (37.1941, 7.8787) centre (38.2548, 8.9393) ccw
  line L54 (39.3155, 10) -> (39.8728, 10)
  arc A62 (41.9941, 7.8787) -> (39.8728, 10) centre (40.9335, 8.9393) ccw
  line L55 (41.9941, 7.8787) -> (41.9941, -7.8787)
  arc A63 (94.6728, -10) -> (96.7941, -7.8787) centre (95.7335, -8.9393) ccw
  line L56 (94.6728, -10) -> (94.1155, -10)
  arc A64 (91.9941, -7.8787) -> (94.1155, -10) centre (93.0548, -8.9393) ccw
  line L57 (91.9941, -7.8787) -> (91.9941, 7.8787)
  arc A65 (94.1155, 10) -> (91.9941, 7.8787) centre (93.0548, 8.9393) ccw
  line L58 (94.1155, 10) -> (94.6728, 10)
  arc A66 (96.7941, 7.8787) -> (94.6728, 10) centre (95.7335, 8.9393) ccw
  line L59 (96.7941, 7.8787) -> (96.7941, -7.8787)
  circle A67 centre (45.4941, -42.5) radius 1.5
  line L60 (-42.1213, -25.5) -> (-109.5263, -25.5)
  arc A68 (-109.5263, -25.5) -> (-110.7763, -25.8349) centre (-109.5263, -28) ccw
  line L61 (-110.7763, -25.8349) -> (-125.9451, -34.5927)
  arc A69 (-125.9451, -34.5927) -> (-127.0931, -37.4646) centre (-124.6951, -36.7577) ccw
  arc A70 (-127.0931, -37.4646) -> (-89.0244, -98.1371) centre (0, 0) ccw
  arc A71 (-89.0244, -98.1371) -> (-85.1797, -97.5355) centre (-87.3447, -96.2855) ccw
  line L62 (-85.1797, -97.5355) -> (-74.6084, -79.2255)
  arc A72 (-71.7106, -78.449) -> (-74.6084, -79.2255) centre (-73.1595, -78.8372) ccw
  line L63 (-71.7106, -78.449) -> (-32.0836, -101.3277)
  arc A73 (-31.3071, -104.2255) -> (-32.0836, -101.3277) centre (-31.6953, -102.7766) ccw
  line L64 (-31.3071, -104.2255) -> (-41.8784, -122.5355)
  arc A74 (-41.8784, -122.5355) -> (-40.477, -126.166) centre (-39.7133, -123.7855) ccw
  arc A75 (-40.477, -126.166) -> (129.5015, -28.0288) centre (0, 0) ccw
  arc A76 (129.5015, -28.0288) -> (127.0581, -25) centre (127.0581, -27.5) ccw
  line L65 (127.0581, -25) -> (105.9155, -25)
  arc A77 (103.7941, -22.8787) -> (105.9155, -25) centre (104.8548, -23.9393) ccw
  line L66 (103.7941, -22.8787) -> (103.7941, 22.8787)
  arc A78 (105.9155, 25) -> (103.7941, 22.8787) centre (104.8548, 23.9393) ccw
  line L67 (105.9155, 25) -> (127.0581, 25)
  arc A79 (127.0581, 25) -> (129.5015, 28.0288) centre (127.0581, 27.5) ccw
  arc A80 (129.5015, 28.0288) -> (-40.477, 126.166) centre (0, 0) ccw
  arc A81 (-40.477, 126.166) -> (-41.8784, 122.5355) centre (-39.7133, 123.7855) ccw
  line L68 (-41.8784, 122.5355) -> (-31.3071, 104.2255)
  arc A82 (-32.0836, 101.3277) -> (-31.3071, 104.2255) centre (-31.6953, 102.7766) ccw
  line L69 (-32.0836, 101.3277) -> (-71.7106, 78.449)
  arc A83 (-74.6084, 79.2255) -> (-71.7106, 78.449) centre (-73.1595, 78.8372) ccw
  line L70 (-74.6084, 79.2255) -> (-85.1797, 97.5355)
  arc A84 (-85.1797, 97.5355) -> (-89.0244, 98.1371) centre (-87.3447, 96.2855) ccw
  arc A85 (-89.0244, 98.1371) -> (-127.0931, 37.4646) centre (0, 0) ccw
  arc A86 (-127.0931, 37.4646) -> (-125.9451, 34.5927) centre (-124.6951, 36.7577) ccw
  line L71 (-125.9451, 34.5927) -> (-110.7763, 25.8349)
  arc A87 (-110.7763, 25.8349) -> (-109.5263, 25.5) centre (-109.5263, 28) ccw
  line L72 (-109.5263, 25.5) -> (-42.1213, 25.5)
  arc A88 (-40, 23.3787) -> (-42.1213, 25.5) centre (-41.0607, 24.4393) ccw
  line L73 (-40, 23.3787) -> (-40, 20.8)
  arc A89 (-40, 20.8) -> (-37.5, 18.3) centre (-37.5, 20.8) ccw
  line L74 (-37.5, 18.3) -> (-34.1213, 18.3)
  arc A90 (-32, 16.1787) -> (-34.1213, 18.3) centre (-33.0607, 17.2393) ccw
  line L75 (-32, 16.1787) -> (-32, -16.1787)
  arc A91 (-34.1213, -18.3) -> (-32, -16.1787) centre (-33.0607, -17.2393) ccw
  line L76 (-34.1213, -18.3) -> (-37.5, -18.3)
  arc A92 (-37.5, -18.3) -> (-40, -20.8) centre (-37.5, -20.8) ccw
  line L77 (-40, -20.8) -> (-40, -23.3787)
  arc A93 (-42.1213, -25.5) -> (-40, -23.3787) centre (-41.0607, -24.4393) ccw
  circle A94 centre (0, 0) radius 3
  circle A95 centre (-94.9024, 87.3758) radius 1.5
  circle A96 centre (123.1209, -38.5) radius 1.5
  circle A97 centre (123.1209, 38.5) radius 1.5
  circle A98 centre (-28.2185, 125.8758) radius 1.5
  circle A99 centre (-94.9024, -87.3758) radius 1.5
  circle A100 centre (-28.2185, -125.8758) radius 1.5
  dimension "d368" = 6
  constraint concentric A0 A94
  measures "d368" diameter of A94
extrude "Extrude12" cut sketch "Sketch9" against normal blind 2 contours A94